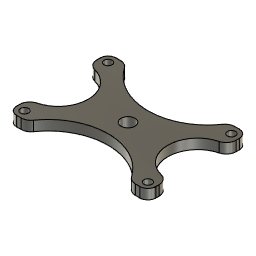
Insta360 One R Mount v4 (Autodesk Fusion 360 design; units mm, degrees)
Autodesk Fusion 360 part; units mm, degrees
sketch "Sketch1" plane through (0, 0, 0) normal (0, 0, 1) x (1, 0, 0)
  line L0 (0, 0) -> (70, 0)
  line L1 (70, 0) -> (70, 50)
  line L2 (70, 50) -> (0, 50)
  line L3 (0, 50) -> (0, 0)
  dimension "d1" = 70
  dimension "d2" = 50
  constraint horizontal L0
  constraint vertical L1
  constraint horizontal L2
  constraint vertical L3
  constraint coincident L0.start L3.end
  measures "d1" distance of L0.start L0.end
  measures "d2" distance of L0.start L2.end
extrude "Extrude1" add sketch "Sketch1" along normal blind 5
sketch "Sketch2" plane through (0, 0, 5) normal (0, 0, 1) x (-1, 0, 0)
  line L0 (0, -50) -> (0, 0)
  line L1 (0, 0) -> (-70, 0)
  line L2 (-70, 0) -> (-70, -50)
  line L3 (-70, -50) -> (0, -50)
  circle A0 centre (-35, -25) radius 3.5
  line L4 (0, -50) -> (-70, 0) construction
  dimension "d5" = 7
  constraint coincident L0.start L3.end
  constraint coincident L1.end L2.start
  constraint midpoint A0.centre L4
  measures "d5" diameter of A0
extrude "Extrude2" cut sketch "Sketch2" against normal blind 5 contours A0
fillet "Fillet1" radius 4 4 edges at (0, 50, 2.5) (0, 0, 2.5) (70, 0, 2.5) (70, 50, 2.5)
sketch "Sketch3" plane through (0, 0, 5) normal (0, 0, 1) x (-1, 0, 0)
  circle A0 centre (-35, -25) radius 3.5
  arc A1 (-70, -46) -> (-66, -50) centre (-66, -46) ccw
  line L0 (-66, -50) -> (-4, -50)
  arc A2 (-4, -50) -> (0, -46) centre (-4, -46) ccw
  line L1 (0, -46) -> (0, -4)
  arc A3 (0, -4) -> (-4, 0) centre (-4, -4) ccw
  line L2 (-4, 0) -> (-66, 0)
  arc A4 (-66, 0) -> (-70, -4) centre (-66, -4) ccw
  line L3 (-70, -4) -> (-70, -46)
  circle A5 centre (-4, -46) radius 2
  dimension "d10" = 4
  dimension "d11" = 4
  dimension "d12" = 4
  measures "d10" diameter of A5
  measures "d11" distance of L0 A2.centre
  measures "d12" distance of L1 A2.centre
extrude "Extrude3" cut sketch "Sketch3" against normal blind 5 contours A5
ref_plane "WorkPlane1" through (35, 25, 2.5) normal (-1, 0, 0) x (0, -1, 0)
ref_plane "WorkPlane2" through (35, 25, 2.5) normal (0, -1, 0) x (1, 0, 0)
mirror "Mirror1" about plane through (35, 25, 2.5) normal (-1, 0, 0) of "Extrude3"
mirror "Mirror2" about plane through (35, 25, 2.5) normal (0, -1, 0) of "Extrude3", "Mirror1"
sketch "Sketch5" plane through (0, 0, 5) normal (0, 0, 1) x (-1, 0, 0)
  circle A0 centre (-66, -4) radius 2
  circle A1 centre (-4, -4) radius 2
  circle A2 centre (-66, -46) radius 2
  circle A3 centre (-4, -46) radius 2
  circle A4 centre (-35, -25) radius 3.5
  arc A5 (-70, -46) -> (-66, -50) centre (-66, -46) ccw
  line L0 (-66, -50) -> (-4, -50)
  arc A6 (-4, -50) -> (0, -46) centre (-4, -46) ccw
  line L1 (0, -46) -> (0, -4)
  arc A7 (0, -4) -> (-4, 0) centre (-4, -4) ccw
  line L2 (-4, 0) -> (-66, 0)
  arc A8 (-66, 0) -> (-70, -4) centre (-66, -4) ccw
  line L3 (-70, -4) -> (-70, -46)
  circle A9 centre (-35, 15) radius 30
  line L4 (-35, -25) -> (-35, 65) construction
  line L5 (-35, -25) -> (102, -25) construction
  circle A10 centre (0, -25) radius 15
  dimension "d19" = 40
  dimension "d20" = 60
  dimension "d21" = 30
  dimension "d22" = 35
  constraint coincident A4.centre L4.start
  constraint vertical L4
  constraint coincident A9.centre L4
  constraint perpendicular L4 L5
  constraint coincident L5 A10.centre
  measures "d19" distance of A9.centre A4.centre
  measures "d20" diameter of A9
  measures "d21" diameter of A10
  measures "d22" distance of A4.centre A10.centre
extrude "Extrude4" cut sketch "Sketch5" against normal blind 5 contours L2 A9 picked at (-36.931, -8.1211)
extrude "Extrude5" cut sketch "Sketch5" against normal blind 5 contours L1 A10 picked at (-3.4009, -21.3347)
mirror "Mirror3" about plane through (35, 25, 2.5) normal (0, -1, 0) of "Extrude4"
mirror "Mirror4" about plane through (35, 25, 2.5) normal (-1, 0, 0) of "Extrude5"
fillet "Fillet2" radius 5 8 edges at (60.9808, 0, 2.5) (70, 10, 2.5) (70, 40, 2.5) (60.9808, 50, 2.5) (9.0192, 50, 2.5) (0, 10, 2.5) (0, 40, 2.5) (9.0192, 0, 2.5)
